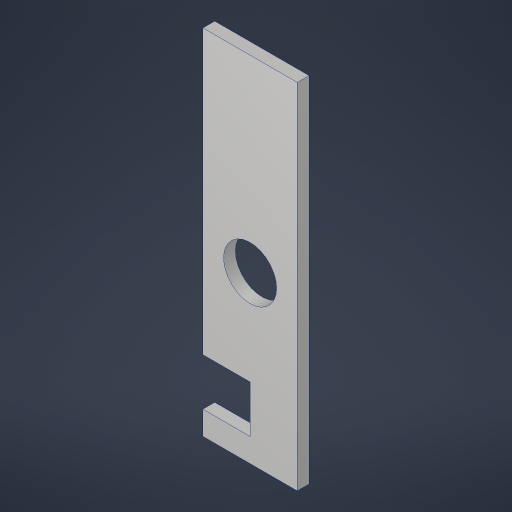
# Autodesk Inventor part: CL6-003
Saved by Autodesk Inventor 2023.4 (Build 274418000, 418)
## iProperties
RuleStatus: InUse
Created: 2025-03-15
Part Number: CL6-003
Material: Aluminum 6061
Document SubType Name: Modeling
Designer: brand
Mass: 132.735 g
Surface Area: 177.419 cm^2
Volume: 49.1612 cm^3
Density: 2.7 g/cm^3
Appearance: Aluminum - Flat
AfterDocNew0: SHOW
AfterDocOpen0: SHOW
Author: brand
Autodesk Inventor part; units mm, degrees
ref_plane "YZ Plane" through (0, 0, 0) normal (1, 0, 0) x (0, 1, 0)
ref_plane "XZ Plane" through (0, 0, 0) normal (0, 1, 0) x (-1, 0, 0)
ref_plane "XY Plane" through (0, 0, 0) normal (0, 0, 1) x (1, 0, 0)
sketch "Sketch1" plane through (0, 0, 0) normal (0, 0, 1) x (1, 0, 0)
  line L0 (-25.4, -95.25) -> (25.4, -95.25)
  line L1 (25.4, -95.25) -> (25.4, 95.25)
  line L2 (25.4, 95.25) -> (-25.4, 95.25)
  line L3 (-25.4, 95.25) -> (-25.4, -95.25)
  line L4 (-25.4, -95.25) -> (25.4, 95.25) construction
  line L5 (25.4, -95.25) -> (-25.4, 95.25) construction
  point P0 (0, 0)
  dimension "width" = 50.8
  dimension "length" = 190.5
  constraints: 12 end point, 2 midpoint, 2 parallel, 1 horizontal, 1 perpendicular
  measures "width" distance of L2.end L1.end
  measures "length" distance of L0.end L1.end
extrude "Extrusion1" add sketch "Sketch1" along normal mid plane 6.35
sketch "Sketch2" plane through (0, 0, 3.175) normal (0, 0, 1) x (1, 0, 0)
  line L0 (-25.4, -95.25) -> (-25.4, 95.25) construction
  line L1 (-25.4, 95.25) -> (25.4, 95.25) construction
  line L2 (25.4, 95.25) -> (25.4, -95.25) construction
  line L3 (25.4, -95.25) -> (-25.4, -95.25) construction
  point P0 (0, 0)
  point P1 (0, -6.35)
  point P2 (0, -95.25)
  dimension "d4" = 88.9
  constraints: 1 midpoint, 1 vertical alignment
  measures "d4" distance from line of L3 point (0, -6.35)
hole "Hole1" at (0, -6.35, 3.175) direction (0, 0, -1) diameter 28.575 end through all
sketch "Sketch3" plane through (0, 0, 3.175) normal (0, 0, 1) x (1, 0, 0)
  circle A0 centre (0, -6.35) radius 14.2875 construction
  line L0 (-25.4, -95.25) -> (-25.4, 95.25) construction
  line L1 (-25.4, 95.25) -> (25.4, 95.25) construction
  line L2 (25.4, 95.25) -> (25.4, -95.25) construction
  line L3 (25.4, -95.25) -> (-25.4, -95.25) construction
  line L4 (-25.4, 95.25) -> (-25.4, -95.25) construction
  line L5 (-25.4, -57.15) -> (0, -57.15)
  line L6 (0, -57.15) -> (0, -82.55)
  line L7 (0, -82.55) -> (-25.4, -82.55)
  line L8 (-25.4, -82.55) -> (-25.4, -57.15)
  point P0 (0, 0)
  dimension "d12" = 25.4
  dimension "d13" = 25.4
  dimension "d14" = 12.7
  constraints: 8 end point, 2 parallel, 1 horizontal, 1 perpendicular, 1 point on line
  measures "d12" distance of L5.start L5.end
  measures "d13" distance of L5.end L6.end
  measures "d14" distance between parallel lines of L3 L7
extrude "Extrusion2" cut sketch "Sketch3" against normal through all
body "Solid1"
